BallJoint 6mm (Autodesk Fusion 360 design; units mm, degrees)
Autodesk Fusion 360 part; units mm, degrees
sketch "Sketch1" plane through (0, 0, 0) normal (0, 0, 1) x (1, 0, 0)
  circle A0 centre (0, 0) radius 3
  circle A1 centre (0, 0) radius 10
  dimension "d1" = 6
  dimension "d2" = 20
  constraint coincident A0.centre A1.centre
  constraint concentric A0 A1
  measures "d1" diameter of A0
  measures "d2" diameter of A1
extrude "Extrude1" add sketch "Sketch1" along normal blind 8 makes body 1
ref_plane "WorkPlane1" through (8, 0, 0) normal (1, 0, 0) x (0, 1, 0)
split "Split1" by plane through (8, 0, 0) normal (1, 0, 0) bodies 1 makes body 2 at (8.25, 5.6514, 5.3333)
ref_plane "WorkPlane2" through (30, 0, 0) normal (1, 0, 0) x (0, 1, 0)
sketch "Sketch2" plane through (30, 0, 0) normal (1, 0, 0) x (0, 1, 0)
  circle A0 centre (0, 4) radius 4
  circle A1 centre (0, 4) radius 3
  dimension "d7" = 8
  dimension "d8" = 6
  constraint coincident origin A0
  constraint concentric A0 A1
  measures "d7" diameter of A0
  measures "d8" diameter of A1
loft "Loft1" add profiles "Sketch2" section 1 face at (8, 2, 2.6667) section 2 on bodies 1 bodies 1
sketch "Sketch3" plane through (30, 0, 0) normal (1, 0, 0) x (0, 1, 0)
  arc A0 (3.3282, 6.2188) -> (-3.3282, 6.2188) centre (0, 4) ccw
  arc A1 (-3.3282, 6.2188) -> (-3.3282, 1.7812) centre (0, 4) ccw
  arc A2 (-3.3282, 1.7812) -> (3.3282, 1.7812) centre (0, 4) ccw
  arc A3 (3.3282, 1.7812) -> (3.3282, 6.2188) centre (0, 4) ccw
  line L0 (0, 0) -> (0, 8) construction
  circle A4 centre (0, 4) radius 3
  dimension "d9" = 6
  constraint coincident L0.start origin
  constraint midpoint A0 L0.end
  constraint concentric A0 A4
  measures "d9" diameter of A4
extrude "Extrude2" cut sketch "Sketch3" against normal blind 17 contours A4 bodies 1
fillet "Fillet1" radius 1.5 2 edges at (-10, 0, 8) (-10, 0, 0) on bodies 1
hidden bodies 2
